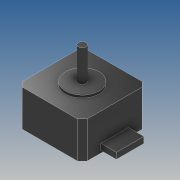
# Autodesk Inventor part: stepper_17HS4023
Saved by Autodesk Inventor 2020 (Build 240168000, 168)
## iProperties
Created: 2021-04-15
Part Number: stepper_17HS4023
Material: Generic
Document SubType Name: Modeling
Designer: stephen
Density: 1 g/cm^3
Appearance: Glossy - Black
Author: stephen
Autodesk Inventor part; units mm, degrees
ref_plane "YZ Plane" through (0, 0, 0) normal (1, 0, 0) x (0, 1, 0)
ref_plane "XZ Plane" through (0, 0, 0) normal (0, 1, 0) x (-1, 0, 0)
ref_plane "XY Plane" through (0, 0, 0) normal (0, 0, 1) x (1, 0, 0)
sketch "Sketch1" plane through (0, 0, 0) normal (0, 1, 0) x (-1, 0, 0)
  line L0 (-18.034, 21.209) -> (18.034, 21.209)
  line L1 (21.209, 18.034) -> (21.209, -18.034)
  line L2 (18.034, -21.209) -> (-18.034, -21.209)
  line L3 (-21.209, -18.034) -> (-21.209, 18.034)
  line L4 (-21.209, 21.209) -> (21.209, -21.209) construction
  line L5 (21.209, 21.209) -> (-21.209, -21.209) construction
  line L6 (21.209, 18.034) -> (18.034, 21.209)
  line L7 (18.034, -21.209) -> (21.209, -18.034)
  line L8 (-18.034, -21.209) -> (-21.209, -18.034)
  line L9 (-21.209, 18.034) -> (-18.034, 21.209)
  point P0 (0, 0)
  dimension "d0" = 42.418
  dimension "d1" = 3.175
  dimension "d2" = 3.175
  dimension "d3" = 3.175
  dimension "d4" = 3.175
  dimension "d5" = 3.175
  dimension "d6" = 3.175
  dimension "d7" = 3.175
  dimension "d8" = 3.175
  constraints: 20 end point, 8 point on line, 2 midpoint, 2 parallel, 2 perpendicular, 1 horizontal
  measures "d0" distance of L5.start L4.end
  measures "d1" distance of L1.start L5.start
  measures "d2" distance of L0.end L5.start
  measures "d3" distance of L2.start L4.end
  measures "d4" distance of L1.end L4.end
  measures "d5" distance of L2.end L5.end
  measures "d6" distance of L3.start L5.end
  measures "d7" distance of L3.end L4.start
  measures "d8" distance of L0.start L4.start
extrude "Extrusion1" add sketch "Sketch1" along normal blind 23.876
sketch "Sketch2" plane through (0, 23.876, 0) normal (0, 1, 0) x (1, 0, 0)
  circle A0 centre (0, 0) radius 10.9982
  dimension "d11" = 21.9964
  constraints: 1 centre point, 1 coincident
  measures "d11" diameter of A0
extrude "Extrusion2" add sketch "Sketch2" along normal blind 1.651
sketch "Sketch3" plane through (0, 25.527, 0) normal (0, 1, 0) x (1, 0, 0)
  circle A0 centre (0, 0) radius 2.4892
  dimension "d14" = 4.9784
  constraints: 1 centre point, 1 coincident
  measures "d14" diameter of A0
extrude "Extrusion3" add sketch "Sketch3" along normal blind 20.828
sketch "Sketch4" plane through (21.209, 0, 18.034) normal (1, 0, 0) x (0, 0, -1)
  line L0 (9.0162, 1.503) -> (27.0518, 1.503)
  line L1 (27.0518, 1.503) -> (27.0518, 5.5109)
  line L2 (27.0518, 5.5109) -> (9.0162, 5.5109)
  line L3 (9.0162, 5.5109) -> (9.0162, 1.503)
  line L4 (9.0162, 1.503) -> (27.0518, 5.5109) construction
  line L5 (27.0518, 1.503) -> (9.0162, 5.5109) construction
  point P0 (18.034, 0)
  point P1 (18.034, 3.5069)
  constraints: 12 end point, 2 midpoint, 2 parallel, 1 horizontal, 1 perpendicular
extrude "Extrusion4" add sketch "Sketch4" along normal blind 10.16
equation "\"d2\" = d1"
equation "\"d3\" = d1"
equation "\"d4\" = d3"
equation "\"d5\" = d1"
equation "\"d6\" = d5"
equation "\"d7\" = d1"
equation "\"d8\" = d7"
body "Solid1"
